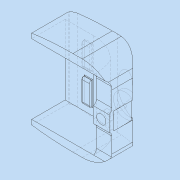
# Autodesk Inventor part: batterybox_back
Saved by Autodesk Inventor 2014 (Build 180170000, 170)
## iProperties
Created: 2014-06-07
Part Number: batterybox_back
Material: Generic
Document SubType Name: Modeling
Designer: brent
Density: 1 g/cm^3
Appearance: Default
Author: brent
Autodesk Inventor part; units mm, degrees
ref_plane "YZ Plane" through (0, 0, 0) normal (1, 0, 0) x (0, 1, 0)
ref_plane "XZ Plane" through (0, 0, 0) normal (0, 1, 0) x (-1, 0, 0)
ref_plane "XY Plane" through (0, 0, 0) normal (0, 0, 1) x (1, 0, 0)
derived "batterybox_sketch.ipt"
sketch "Sketch1" plane through (0, 0, 0) normal (1, 0, 0) x (0, 1, 0)
  line L0 (-14, 0) -> (14, 0)
  line L1 (-57, 0) -> (57.7, 0)
  line L2 (57.7, 0) -> (57.7, -55)
  line L3 (57.7, -55) -> (-57, -55)
  line L4 (-57, -55) -> (-57, 0)
  line L5 (-69.7, 0) -> (70.4, 0)
  line L6 (70.4, 0) -> (70.4, -64.525)
  line L7 (70.4, -64.525) -> (-69.7, -64.525)
  line L8 (-69.7, -64.525) -> (-69.7, 0)
  point P0 (0, 0)
extrude "Extrusion1" add sketch "Sketch1" along normal blind 101.6 contours L4 L3 L2 L5 L6 L7 L8
sketch "Sketch2" plane through (0, -57, -55) normal (0, 0, 1) x (1, 0, 0)
  line L0 (0, 0) -> (0, 114.7) projected
  line L1 (0, 0) -> (101.6, 0) projected
  line L2 (0, 114.7) -> (101.6, 114.7) projected
  line L3 (31.75, 114.7) -> (44.45, 114.7)
  line L4 (44.45, 114.7) -> (44.45, 0)
  line L5 (44.45, 0) -> (31.75, 0)
  line L6 (31.75, 0) -> (31.75, 114.7)
  point P0 (0, 57)
  dimension "d4" = 31.75
  dimension "d14" = 12.7
  constraints: 8 end point, 2 parallel, 2 point on line, 1 horizontal, 1 perpendicular
  measures "d4" distance between parallel lines of L0 L6
  measures "d14" distance between parallel lines of L6 L4
extrude "Extrusion2" add sketch "Sketch2" along normal blind 4.7625 contours L6 L2 L4 L1
sketch "Sketch3" plane through (31.75, -57, -55) normal (-1, 0, 0) x (0, 0, 1)
  line L0 (0, 0) -> (0, 114.7) projected
  line L1 (4.7625, 0) -> (0, 0) projected
  line L2 (4.7625, 114.7) -> (4.7625, 0) projected
  line L3 (0, 114.7) -> (4.7625, 114.7) projected
  line L4 (0, 63.7) -> (4.7625, 63.7)
  line L5 (4.7625, 63.7) -> (4.7625, 51)
  line L6 (4.7625, 51) -> (0, 51)
  line L7 (0, 51) -> (0, 63.7)
  line L8 (0, 0) -> (4.7625, 0)
  line L9 (4.7625, 0) -> (4.7625, 12.7)
  line L10 (4.7625, 12.7) -> (0, 12.7)
  line L11 (0, 12.7) -> (0, 0)
  line L12 (0, 114.7) -> (4.7625, 114.7)
  line L13 (4.7625, 114.7) -> (4.7625, 102)
  line L14 (4.7625, 102) -> (0, 102)
  line L15 (0, 102) -> (0, 114.7)
  point P0 (55, 57)
  dimension "d7" = 114.7
  dimension "d8" = 51
  dimension "d9" = 51
  dimension "d10" = 12.7
  dimension "d11" = 12.7
  constraints: 24 end point, 6 parallel, 4 point on line, 3 horizontal, 3 perpendicular
  measures "d7" distance between parallel lines of L3 L1
  measures "d8" distance between parallel lines of L3 L4
  measures "d9" distance between parallel lines of L1 L6
  measures "d10" distance of L9.end L8.end
  measures "d11" distance between parallel lines of L12 L14
extrude "Extrusion3" cut sketch "Sketch3" against normal through all contours L0 L10 L2 L1 | L0 L4 L2 L6 | L0 L3 L2 L14
fillet "Fillet1" radius 0.7937 2 edges at (44.45, -25.15, -55) (44.45, 25.85, -55)
fillet "Fillet1" radius 0.7937 12 edges at (31.75, 25.85, -55) (31.75, -25.15, -55) (38.1, 6.7, -55) (38.1, -6, -55) (38.1, -44.3, -55) (38.1, 45, -55) (31.75, 6.7, -52.6187) (31.75, 45, -52.6187) (31.75, -6, -52.6187) (31.75, -44.3, -52.6188) (31.75, 25.85, -50.2375) (31.75, -25.15, -50.2375)
fillet "Fillet1" radius 3.175 4 edges at (38.1, -6, -50.2375) (38.1, -44.3, -50.2375) (38.1, 6.7, -50.2375) (38.1, 45, -50.2375)
sketch "Sketch4" plane through (101.6, -69.7, -64.525) normal (1, 0, 0) x (0, 0, -1)
  line L0 (-64.525, 140.1) -> (0, 140.1)
  line L1 (0, 140.1) -> (0, 0)
  line L2 (0, 0) -> (-64.525, 0)
  line L3 (-64.525, 0) -> (-64.525, 140.1)
  point P0 (-64.525, 69.7)
  constraints: 8 end point, 2 parallel, 1 horizontal, 1 perpendicular
extrude "Extrusion4" add sketch "Sketch4" along normal blind 25.4
sketch "Sketch7" plane through (0, -69.7, 0) normal (0, 0, 1) x (1, 0, 0)
  line L0 (0, 0) -> (127, 0) projected
  line L1 (0, 140.1) -> (127, 140.1) projected
  line L2 (101.6, 127.4) -> (101.6, 12.7) projected
  circle A0 centre (114.3, 70.05) radius 2.5527
  point P0 (0, 69.7)
  dimension "d41" = 5.1054
  dimension "d42" = 12.7
  dimension "d43" = 140.1
  dimension "d44" = 70.05
  constraints: 1 centre point
  measures "d41" diameter of A0
  measures "d42" distance from line of L2 A0.centre
  measures "d43" distance between parallel lines of L0 L1
  measures "d44" distance from line of L0 A0.centre
extrude "Extrusion7" cut sketch "Sketch7" against normal through all
sketch "Sketch8" plane through (0, -69.7, 0) normal (0, 0, 1) x (1, 0, 0)
  circle A0 centre (114.3, 70.05) radius 2.5527 projected
  circle A1 centre (114.3, 70.05) radius 7.62
  point P0 (0, 69.7)
  dimension "d47" = 15.24
  constraints: 1 centre point, 1 coincident
  measures "d47" diameter of A1
extrude "Extrusion8" cut sketch "Sketch8" against normal blind 12.7
chamfer "Chamfer5" distance 26.9875 angle 45 1 edges at (101.6, 0.35, -55)
sketch "Sketch9" plane through (0, -69.7, -64.525) normal (0, 0, -1) x (-1, 0, 0)
  circle A0 centre (-114.3, 70.05) radius 2.5527 projected
  circle A1 centre (-114.3, 70.05) radius 19.05
  point P0 (0, 69.7)
  dimension "d50" = 38.1
  constraints: 1 centre point, 1 coincident
  measures "d50" diameter of A1
extrude "Extrusion9" cut sketch "Sketch9" against normal blind 25.4
chamfer "Chamfer12" distance 25.4 angle 45 2 edges at (127, 42.4745, -64.525) (127, -41.7745, -64.525)
sketch "Sketch23" plane through (0, -69.7, 0) normal (0, 0, 1) x (1, 0, 0)
  circle A0 centre (114.3, 70.05) radius 7.62 projected
  line L0 (101.6, 12.7) -> (0, 12.7) projected
  line L1 (0, 12.7) -> (0, 0) projected
  line L2 (0, 0) -> (127, 0) projected
  line L3 (127, 140.1) -> (127, 0) projected
  line L4 (0, 140.1) -> (127, 140.1) projected
  line L5 (0, 140.1) -> (0, 127.4) projected
  line L6 (0, 127.4) -> (101.6, 127.4) projected
  line L7 (101.6, 127.4) -> (101.6, 12.7) projected
  line L8 (101.6, 127.4) -> (127, 127.4)
  line L9 (127, 127.4) -> (127, 82.75)
  line L10 (127, 82.75) -> (101.6, 82.75)
  line L11 (101.6, 82.75) -> (101.6, 127.4)
  line L12 (101.6, 12.7) -> (127, 12.7)
  line L13 (127, 12.7) -> (127, 57.35)
  line L14 (127, 57.35) -> (101.6, 57.35)
  line L15 (101.6, 57.35) -> (101.6, 12.7)
  point P0 (0, 69.7)
  dimension "d170" = 12.7
  dimension "d171" = 12.7
  constraints: 16 end point, 4 parallel, 2 horizontal, 2 perpendicular, 2 point on line
  measures "d170" distance from line of A0.centre L14
  measures "d171" distance from line of L10 A0.centre
extrude "Extrusion23" cut sketch "Sketch23" against normal blind 4.7625 contours L7 L14 L3 L12 | L7 L8 L3 L10
chamfer "Chamfer13" distance 19.05 angle 45 2 edges at (127, -69.7, -19.5625) (127, 70.4, -19.5625)
chamfer "Chamfer14" distance 19.05 angle 45 1 edges at (95.25, 0.35, -64.525)
fillet "Fillet23" radius 7.9375 4 edges at (114.3, -12.35, -4.7625) (114.3, 13.05, -4.7625) (111.125, 57.7, -4.7625) (111.125, -57, -4.7625)
chamfer "Chamfer16" distance 2.54 angle 45 1 edges at (127, 0.35, -39.125)
fillet "Fillet24" radius 190.5 1 edges at (127, 0.35, -36.585)
chamfer "Chamfer17" distance 4.7625 angle 45 3 edges at (0, 0.35, -64.525) (0, 70.4, -32.2625) (0, -69.7, -32.2625)
fillet "Fillet25" radius 484.1875 2 edges at (4.7625, 70.4, -32.2625) (4.7625, -69.7, -32.2625)
fillet "Fillet26" radius 60.325 2 edges at (107.95, -69.7, -29.0875) (107.95, 70.4, -29.0875)
fillet "Fillet27" radius 60.325 2 edges at (101.6, -51.1599, -64.525) (101.6, 51.8599, -64.525)
fillet "Fillet28" radius 12.7 2 edges at (127, 51.35, -21.9167) (127, -50.65, -21.9167)
fillet "Fillet29" radius 12.7 1 edges at (4.7625, 0.35, -64.525)
fillet "Fillet30" radius 68.2625 1 edges at (74.6125, 0.35, -55)
fillet "Fillet31" radius 68.2625 1 edges at (101.6, 0.35, -28.0125)
equation "\"d44\" = 0.5 * d43"
body "Solid1"
